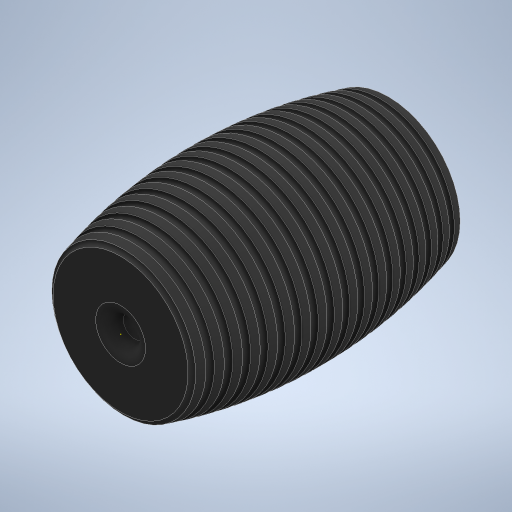
# Autodesk Inventor part: roller-5
Saved by Autodesk Inventor 2024.2 (Build 282272000, 272)
## iProperties
Created: 2024-04-23
Part Number: roller-5
Material: Rubber
Document SubType Name: Modeling
Designer: Robin
Density: 0.93 g/cm^3
Appearance: Rubber - Black
Author: Robin
Autodesk Inventor part; units mm, degrees
ref_plane "YZ Plane" through (0, 0, 0) normal (1, 0, 0) x (0, 1, 0)
ref_plane "XZ Plane" through (0, 0, 0) normal (0, 1, 0) x (-1, 0, 0)
ref_plane "XY Plane" through (0, 0, 0) normal (0, 0, 1) x (1, 0, 0)
sketch "Sketch1" plane through (0, 0, 0) normal (0, 1, 0) x (-1, 0, 0)
  line L0 (6.5, 9.75) -> (0, 9.75)
  line L1 (0, 9.75) -> (0, -9.75)
  line L2 (0, -9.75) -> (6.5, -9.75)
  line L3 (6.5, -9.75) -> (6.5, 9.75)
  line L4 (0.8, 9.75) -> (0.8, -9.75)
  arc A0 (5.114543, -9.75) -> (5.114543, 9.75) centre (-28.5, 0) ccw
  circle A1 centre (6.5, 0) radius 0.25
  circle A2 centre (6.48273, 1.099377) radius 0.25
  circle A3 centre (6.430935, 2.197668) radius 0.25
  circle A4 centre (6.344669, 3.293791) radius 0.25
  circle A5 centre (6.224015, 4.386663) radius 0.25
  circle A6 centre (6.069092, 5.475206) radius 0.25
  circle A7 centre (5.880054, 6.558346) radius 0.25
  circle A8 centre (5.657087, 7.635013) radius 0.25
  circle A9 centre (5.400411, 8.704146) radius 0.25
  circle A10 centre (5.110279, 9.764689) radius 0.25
  circle A11 centre (4.786978, 10.815595) radius 0.25
  circle A12 centre (4.430827, 11.855827) radius 0.25
  circle A13 centre (4.042177, 12.884359) radius 0.25
  circle A14 centre (3.621412, 13.900176) radius 0.25
  circle A15 centre (3.168947, 14.902275) radius 0.25
  circle A16 centre (2.685228, 15.889667) radius 0.25
  circle A17 centre (2.170734, 16.861379) radius 0.25
  circle A18 centre (1.625971, 17.81645) radius 0.25
  circle A19 centre (1.051477, 18.753938) radius 0.25
  circle A20 centre (0.44782, 19.672918) radius 0.25
  circle A21 centre (-0.184405, 20.572484) radius 0.25
  circle A22 centre (-0.844575, 21.451747) radius 0.25
  circle A23 centre (-1.532037, 22.30984) radius 0.25
  circle A24 centre (-2.246113, 23.145915) radius 0.25
  circle A25 centre (-2.986098, 23.959149) radius 0.25
  circle A26 centre (-3.751263, 24.748737) radius 0.25
  circle A27 centre (-4.540851, 25.513902) radius 0.25
  circle A28 centre (-5.354085, 26.253887) radius 0.25
  circle A29 centre (-6.19016, 26.967963) radius 0.25
  circle A30 centre (-7.048253, 27.655425) radius 0.25
  circle A31 centre (-7.927516, 28.315595) radius 0.25
  circle A32 centre (-8.827082, 28.94782) radius 0.25
  circle A33 centre (-9.746062, 29.551477) radius 0.25
  circle A34 centre (-10.68355, 30.125971) radius 0.25
  circle A35 centre (-11.638621, 30.670734) radius 0.25
  circle A36 centre (-12.610333, 31.185228) radius 0.25
  circle A37 centre (-13.597725, 31.668947) radius 0.25
  circle A38 centre (-14.599824, 32.121412) radius 0.25
  circle A39 centre (-15.615641, 32.542177) radius 0.25
  circle A40 centre (-16.644173, 32.930827) radius 0.25
  circle A41 centre (-17.684405, 33.286978) radius 0.25
  circle A42 centre (-18.735311, 33.610279) radius 0.25
  circle A43 centre (-19.795854, 33.900411) radius 0.25
  circle A44 centre (-20.864987, 34.157087) radius 0.25
  circle A45 centre (-21.941654, 34.380054) radius 0.25
  circle A46 centre (-23.024794, 34.569092) radius 0.25
  circle A47 centre (-24.113337, 34.724015) radius 0.25
  circle A48 centre (-25.206209, 34.844669) radius 0.25
  circle A49 centre (-26.302332, 34.930935) radius 0.25
  circle A50 centre (-27.400623, 34.98273) radius 0.25
  circle A51 centre (-28.5, 35) radius 0.25
  circle A52 centre (-29.599377, 34.98273) radius 0.25
  circle A53 centre (-30.697668, 34.930935) radius 0.25
  circle A54 centre (-31.793791, 34.844669) radius 0.25
  circle A55 centre (-32.886663, 34.724015) radius 0.25
  circle A56 centre (-33.975206, 34.569092) radius 0.25
  circle A57 centre (-35.058346, 34.380054) radius 0.25
  circle A58 centre (-36.135013, 34.157087) radius 0.25
  circle A59 centre (-37.204146, 33.900411) radius 0.25
  circle A60 centre (-38.264689, 33.610279) radius 0.25
  circle A61 centre (-39.315595, 33.286978) radius 0.25
  circle A62 centre (-40.355827, 32.930827) radius 0.25
  circle A63 centre (-41.384359, 32.542177) radius 0.25
  circle A64 centre (-42.400176, 32.121412) radius 0.25
  circle A65 centre (-43.402275, 31.668947) radius 0.25
  circle A66 centre (-44.389667, 31.185228) radius 0.25
  circle A67 centre (-45.361379, 30.670734) radius 0.25
  circle A68 centre (-46.31645, 30.125971) radius 0.25
  circle A69 centre (-47.253938, 29.551477) radius 0.25
  circle A70 centre (-48.172918, 28.94782) radius 0.25
  circle A71 centre (-49.072484, 28.315595) radius 0.25
  circle A72 centre (-49.951747, 27.655425) radius 0.25
  circle A73 centre (-50.80984, 26.967963) radius 0.25
  circle A74 centre (-51.645915, 26.253887) radius 0.25
  circle A75 centre (-52.459149, 25.513902) radius 0.25
  circle A76 centre (-53.248737, 24.748737) radius 0.25
  circle A77 centre (-54.013902, 23.959149) radius 0.25
  circle A78 centre (-54.753887, 23.145915) radius 0.25
  circle A79 centre (-55.467963, 22.30984) radius 0.25
  circle A80 centre (-56.155425, 21.451747) radius 0.25
  circle A81 centre (-56.815595, 20.572484) radius 0.25
  circle A82 centre (-57.44782, 19.672918) radius 0.25
  circle A83 centre (-58.051477, 18.753938) radius 0.25
  circle A84 centre (-58.625971, 17.81645) radius 0.25
  circle A85 centre (-59.170734, 16.861379) radius 0.25
  circle A86 centre (-59.685228, 15.889667) radius 0.25
  circle A87 centre (-60.168947, 14.902275) radius 0.25
  circle A88 centre (-60.621412, 13.900176) radius 0.25
  circle A89 centre (-61.042177, 12.884359) radius 0.25
  circle A90 centre (-61.430827, 11.855827) radius 0.25
  circle A91 centre (-61.786978, 10.815595) radius 0.25
  circle A92 centre (-62.110279, 9.764689) radius 0.25
  circle A93 centre (-62.400411, 8.704146) radius 0.25
  circle A94 centre (-62.657087, 7.635013) radius 0.25
  circle A95 centre (-62.880054, 6.558346) radius 0.25
  circle A96 centre (-63.069092, 5.475206) radius 0.25
  circle A97 centre (-63.224015, 4.386663) radius 0.25
  circle A98 centre (-63.344669, 3.293791) radius 0.25
  circle A99 centre (-63.430935, 2.197668) radius 0.25
  circle A100 centre (-63.48273, 1.099377) radius 0.25
  circle A101 centre (-63.5, 0) radius 0.25
  circle A102 centre (-63.48273, -1.099377) radius 0.25
  circle A103 centre (-63.430935, -2.197668) radius 0.25
  circle A104 centre (-63.344669, -3.293791) radius 0.25
  circle A105 centre (-63.224015, -4.386663) radius 0.25
  circle A106 centre (-63.069092, -5.475206) radius 0.25
  circle A107 centre (-62.880054, -6.558346) radius 0.25
  circle A108 centre (-62.657087, -7.635013) radius 0.25
  circle A109 centre (-62.400411, -8.704146) radius 0.25
  circle A110 centre (-62.110279, -9.764689) radius 0.25
  circle A111 centre (-61.786978, -10.815595) radius 0.25
  circle A112 centre (-61.430827, -11.855827) radius 0.25
  circle A113 centre (-61.042177, -12.884359) radius 0.25
  circle A114 centre (-60.621412, -13.900176) radius 0.25
  circle A115 centre (-60.168947, -14.902275) radius 0.25
  circle A116 centre (-59.685228, -15.889667) radius 0.25
  circle A117 centre (-59.170734, -16.861379) radius 0.25
  circle A118 centre (-58.625971, -17.81645) radius 0.25
  circle A119 centre (-58.051477, -18.753938) radius 0.25
  circle A120 centre (-57.44782, -19.672918) radius 0.25
  circle A121 centre (-56.815595, -20.572484) radius 0.25
  circle A122 centre (-56.155425, -21.451747) radius 0.25
  circle A123 centre (-55.467963, -22.30984) radius 0.25
  circle A124 centre (-54.753887, -23.145915) radius 0.25
  circle A125 centre (-54.013902, -23.959149) radius 0.25
  circle A126 centre (-53.248737, -24.748737) radius 0.25
  circle A127 centre (-52.459149, -25.513902) radius 0.25
  circle A128 centre (-51.645915, -26.253887) radius 0.25
  circle A129 centre (-50.80984, -26.967963) radius 0.25
  circle A130 centre (-49.951747, -27.655425) radius 0.25
  circle A131 centre (-49.072484, -28.315595) radius 0.25
  circle A132 centre (-48.172918, -28.94782) radius 0.25
  circle A133 centre (-47.253938, -29.551477) radius 0.25
  circle A134 centre (-46.31645, -30.125971) radius 0.25
  circle A135 centre (-45.361379, -30.670734) radius 0.25
  circle A136 centre (-44.389667, -31.185228) radius 0.25
  circle A137 centre (-43.402275, -31.668947) radius 0.25
  circle A138 centre (-42.400176, -32.121412) radius 0.25
  circle A139 centre (-41.384359, -32.542177) radius 0.25
  circle A140 centre (-40.355827, -32.930827) radius 0.25
  circle A141 centre (-39.315595, -33.286978) radius 0.25
  circle A142 centre (-38.264689, -33.610279) radius 0.25
  circle A143 centre (-37.204146, -33.900411) radius 0.25
  circle A144 centre (-36.135013, -34.157087) radius 0.25
  circle A145 centre (-35.058346, -34.380054) radius 0.25
  circle A146 centre (-33.975206, -34.569092) radius 0.25
  circle A147 centre (-32.886663, -34.724015) radius 0.25
  circle A148 centre (-31.793791, -34.844669) radius 0.25
  circle A149 centre (-30.697668, -34.930935) radius 0.25
  circle A150 centre (-29.599377, -34.98273) radius 0.25
  circle A151 centre (-28.5, -35) radius 0.25
  circle A152 centre (-27.400623, -34.98273) radius 0.25
  circle A153 centre (-26.302332, -34.930935) radius 0.25
  circle A154 centre (-25.206209, -34.844669) radius 0.25
  circle A155 centre (-24.113337, -34.724015) radius 0.25
  circle A156 centre (-23.024794, -34.569092) radius 0.25
  circle A157 centre (-21.941654, -34.380054) radius 0.25
  circle A158 centre (-20.864987, -34.157087) radius 0.25
  circle A159 centre (-19.795854, -33.900411) radius 0.25
  circle A160 centre (-18.735311, -33.610279) radius 0.25
  circle A161 centre (-17.684405, -33.286978) radius 0.25
  circle A162 centre (-16.644173, -32.930827) radius 0.25
  circle A163 centre (-15.615641, -32.542177) radius 0.25
  circle A164 centre (-14.599824, -32.121412) radius 0.25
  circle A165 centre (-13.597725, -31.668947) radius 0.25
  circle A166 centre (-12.610333, -31.185228) radius 0.25
  circle A167 centre (-11.638621, -30.670734) radius 0.25
  circle A168 centre (-10.68355, -30.125971) radius 0.25
  circle A169 centre (-9.746062, -29.551477) radius 0.25
  circle A170 centre (-8.827082, -28.94782) radius 0.25
  circle A171 centre (-7.927516, -28.315595) radius 0.25
  circle A172 centre (-7.048253, -27.655425) radius 0.25
  circle A173 centre (-6.19016, -26.967963) radius 0.25
  circle A174 centre (-5.354085, -26.253887) radius 0.25
  circle A175 centre (-4.540851, -25.513902) radius 0.25
  circle A176 centre (-3.751263, -24.748737) radius 0.25
  circle A177 centre (-2.986098, -23.959149) radius 0.25
  circle A178 centre (-2.246113, -23.145915) radius 0.25
  circle A179 centre (-1.532037, -22.30984) radius 0.25
  circle A180 centre (-0.844575, -21.451747) radius 0.25
  circle A181 centre (-0.184405, -20.572484) radius 0.25
  circle A182 centre (0.44782, -19.672918) radius 0.25
  circle A183 centre (1.051477, -18.753938) radius 0.25
  circle A184 centre (1.625971, -17.81645) radius 0.25
  circle A185 centre (2.170734, -16.861379) radius 0.25
  circle A186 centre (2.685228, -15.889667) radius 0.25
  circle A187 centre (3.168947, -14.902275) radius 0.25
  circle A188 centre (3.621412, -13.900176) radius 0.25
  circle A189 centre (4.042177, -12.884359) radius 0.25
  circle A190 centre (4.430827, -11.855827) radius 0.25
  circle A191 centre (4.786978, -10.815595) radius 0.25
  circle A192 centre (5.110279, -9.764689) radius 0.25
  circle A193 centre (5.400411, -8.704146) radius 0.25
  circle A194 centre (5.657087, -7.635013) radius 0.25
  circle A195 centre (5.880054, -6.558346) radius 0.25
  circle A196 centre (6.069092, -5.475206) radius 0.25
  circle A197 centre (6.224015, -4.386663) radius 0.25
  circle A198 centre (6.344669, -3.293791) radius 0.25
  circle A199 centre (6.430935, -2.197668) radius 0.25
  circle A200 centre (6.48273, -1.099377) radius 0.25
  point P0 (0, 0)
  point P1 (6.473985, -1.349224)
  point P2 (6.48969, -0.849473)
  point P3 (6.499107, -0.249998)
  point P4 (6.499107, 0.249998)
  point P5 (6.48969, 0.849473)
  point P6 (6.473985, 1.349224)
  point P7 (6.445742, 1.948107)
  point P8 (6.414347, 2.447117)
  point P9 (6.367307, 3.044818)
  point P10 (6.320253, 3.542596)
  point P11 (6.254462, 4.138524)
  point P12 (6.191796, 4.634578)
  point P13 (6.107318, 5.228146)
  point P14 (6.029102, 5.721987)
  point P15 (5.926022, 6.312608)
  point P16 (5.832332, 6.803749)
  point P17 (5.710751, 7.390841)
  point P18 (5.60168, 7.878796)
  point P19 (5.461718, 8.46178)
  point P20 (5.337374, 8.946068)
  point P21 (5.179169, 9.524368)
  point P22 (4.860711, 9.75)
  point P23 (4.860711, -9.75)
  point P24 (5.179169, -9.524368)
  point P25 (5.337374, -8.946068)
  point P26 (5.461718, -8.46178)
  point P27 (5.60168, -7.878796)
  point P28 (5.710751, -7.390841)
  point P29 (5.832332, -6.803749)
  point P30 (5.926022, -6.312608)
  point P31 (6.029102, -5.721987)
  point P32 (6.107318, -5.228146)
  point P33 (6.191796, -4.634578)
  point P34 (6.254462, -4.138524)
  point P35 (6.320253, -3.542596)
  point P36 (6.367307, -3.044818)
  point P37 (6.414347, -2.447117)
  point P38 (6.445742, -1.948107)
  point P39 (6.5, -0.849974)
  point P40 (6.5, -1.348779)
  point P41 (6.5, -1.957397)
  point P42 (6.5, -2.437939)
  point P43 (6.5, -3.097903)
  point P44 (6.5, -3.489679)
  point P45 (5.359847, -9.75)
  point P46 (6.5, -0.25)
  point P47 (5.359847, 9.75)
  point P48 (6.5, 3.489679)
  point P49 (6.5, 3.097903)
  point P50 (6.5, 2.437939)
  point P51 (6.5, 1.957397)
  point P52 (6.5, 1.348779)
  point P53 (6.5, 0.849974)
  point P54 (6.5, 0.25)
  dimension "d3" = 35
  dimension "d0" = 6.5
  dimension "d1" = 19.5
  dimension "d2" = 0.8
  dimension "d5" = 0.5
  dimension "d8" = 360
  constraints: 200 centre point, 10 end point, 4 point on line, 2 parallel, 2 perpendicular, 2 vertical alignment, 1 coincident, 1 horizontal, 1 horizontal alignment, 1 midpoint, 406 other
  measures "d0" distance of L1.end L2.end
  measures "d1" distance of L2.end L0.start
  measures "d2" distance between parallel lines of L1 L4
  measures "d5" diameter of A1
sketch "Sketch1 outline for Revolution1" plane through (0, 0, 0) normal (0, 1, 0) x (-1, 0, 0)
  arc A0 (6.473985, -1.349224) -> (6.48969, -0.849473) centre (6.48273, -1.099377) cw
  arc A1 (6.445742, -1.948107) -> (6.473985, -1.349224) centre (-28.5, 0) ccw
  arc A2 (6.414347, -2.447117) -> (6.445742, -1.948107) centre (6.430935, -2.197668) cw
  arc A3 (6.367307, -3.044818) -> (6.414347, -2.447117) centre (-28.5, 0) ccw
  arc A4 (6.320253, -3.542596) -> (6.367307, -3.044818) centre (6.344669, -3.293791) cw
  arc A5 (6.254462, -4.138524) -> (6.320253, -3.542596) centre (-28.5, 0) ccw
  arc A6 (6.191796, -4.634578) -> (6.254462, -4.138524) centre (6.224015, -4.386663) cw
  arc A7 (6.107318, -5.228146) -> (6.191796, -4.634578) centre (-28.5, 0) ccw
  arc A8 (6.029102, -5.721987) -> (6.107318, -5.228146) centre (6.069092, -5.475206) cw
  arc A9 (5.926022, -6.312608) -> (6.029102, -5.721987) centre (-28.5, 0) ccw
  arc A10 (5.832332, -6.803749) -> (5.926022, -6.312608) centre (5.880054, -6.558346) cw
  arc A11 (5.710751, -7.390841) -> (5.832332, -6.803749) centre (-28.5, 0) ccw
  arc A12 (5.60168, -7.878796) -> (5.710751, -7.390841) centre (5.657087, -7.635013) cw
  arc A13 (5.461718, -8.46178) -> (5.60168, -7.878796) centre (-28.5, 0) ccw
  arc A14 (5.337374, -8.946068) -> (5.461718, -8.46178) centre (5.400411, -8.704146) cw
  arc A15 (5.179169, -9.524368) -> (5.337374, -8.946068) centre (-28.5, 0) ccw
  arc A16 (4.860711, -9.75) -> (5.179169, -9.524368) centre (5.110279, -9.764689) cw
  line L0 (0.8, -9.75) -> (4.860711, -9.75)
  line L1 (0.8, 9.75) -> (0.8, -9.75)
  line L2 (4.860711, 9.75) -> (0.8, 9.75)
  arc A17 (5.179169, 9.524368) -> (4.860711, 9.75) centre (5.110279, 9.764689) cw
  arc A18 (5.337374, 8.946068) -> (5.179169, 9.524368) centre (-28.5, 0) ccw
  arc A19 (5.461718, 8.46178) -> (5.337374, 8.946068) centre (5.400411, 8.704146) cw
  arc A20 (5.60168, 7.878796) -> (5.461718, 8.46178) centre (-28.5, 0) ccw
  arc A21 (5.710751, 7.390841) -> (5.60168, 7.878796) centre (5.657087, 7.635013) cw
  arc A22 (5.832332, 6.803749) -> (5.710751, 7.390841) centre (-28.5, 0) ccw
  arc A23 (5.926022, 6.312608) -> (5.832332, 6.803749) centre (5.880054, 6.558346) cw
  arc A24 (6.029102, 5.721987) -> (5.926022, 6.312608) centre (-28.5, 0) ccw
  arc A25 (6.107318, 5.228146) -> (6.029102, 5.721987) centre (6.069092, 5.475206) cw
  arc A26 (6.191796, 4.634578) -> (6.107318, 5.228146) centre (-28.5, 0) ccw
  arc A27 (6.254462, 4.138524) -> (6.191796, 4.634578) centre (6.224015, 4.386663) cw
  arc A28 (6.320253, 3.542596) -> (6.254462, 4.138524) centre (-28.5, 0) ccw
  arc A29 (6.367307, 3.044818) -> (6.320253, 3.542596) centre (6.344669, 3.293791) cw
  arc A30 (6.414347, 2.447117) -> (6.367307, 3.044818) centre (-28.5, 0) ccw
  arc A31 (6.445742, 1.948107) -> (6.414347, 2.447117) centre (6.430935, 2.197668) cw
  arc A32 (6.473985, 1.349224) -> (6.445742, 1.948107) centre (-28.5, 0) ccw
  arc A33 (6.48969, 0.849473) -> (6.473985, 1.349224) centre (6.48273, 1.099377) cw
  arc A34 (6.499107, 0.249998) -> (6.48969, 0.849473) centre (-28.5, 0) ccw
  arc A35 (6.499107, -0.249998) -> (6.499107, 0.249998) centre (6.5, 0) cw
  arc A36 (6.48969, -0.849473) -> (6.499107, -0.249998) centre (-28.5, 0) ccw
revolve "Revolution1" add sketch "Sketch1 outline for Revolution1" angle 360 about axis through (0, 0, 9.75) along (0, 0, -1)
sketch "Sketch4" plane through (0, 0, 9.75) normal (0, 0, 1) x (1, 0, 0)
  point P0 (0, 0)
fillet "Fillet1" radius 1 1 edges at (0.8, 0, 9.75)
fillet "Fillet2" radius 1 1 edges at (0.8, 0, -9.75)
body "Solid1"
